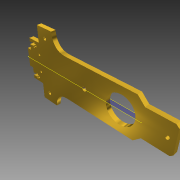
# Autodesk Inventor part: tiltColumnStepperSide02_RB01
Saved by Autodesk Inventor 2013 (Build 170138000, 138)
## iProperties
Created: 2014-06-14
Part Number: tiltColumnStepperSide02_RB01
Material: Gold
Document SubType Name: Modeling
Designer: Byron
Density: 19.3 g/cm^3
Mass: 1131.92 g
Surface Area: 227.905 cm^2
Volume: 58.6488 cm^3
Author: Byron
Autodesk Inventor part; units mm, degrees
ref_plane "YZ Plane" through (0, 0, 0) normal (1, 0, 0) x (0, 1, 0)
ref_plane "XZ Plane" through (0, 0, 0) normal (0, 1, 0) x (-1, 0, 0)
ref_plane "XY Plane" through (0, 0, 0) normal (0, 0, 1) x (1, 0, 0)
sketch "Sketch1" plane through (0, 0, 0) normal (0, 0, 1) x (1, 0, 0)
  line L0 (-21.15, 15.4985) -> (-15.4985, 21.15)
  line L1 (-15.4985, 21.15) -> (15.4985, 21.15)
  line L2 (15.4985, 21.15) -> (21.15, 15.4985)
  line L3 (21.15, 15.4985) -> (21.15, -15.4985)
  line L4 (21.15, -15.4985) -> (15.4985, -21.15)
  line L5 (15.4985, -21.15) -> (-15.4985, -21.15)
  line L6 (-15.4985, -21.15) -> (-21.15, -15.4985)
  line L7 (-21.15, -15.4985) -> (-21.15, 15.4985)
  line L8 (28.575, -18.574) -> (28.575, 18.574)
  line L9 (28.575, 18.574) -> (18.574, 28.575)
  line L10 (18.574, 28.575) -> (-18.574, 28.575)
  line L11 (-18.574, 28.575) -> (-28.575, 18.574)
  line L12 (-28.575, 18.574) -> (-28.575, -18.574)
  line L13 (-28.575, -18.574) -> (-18.574, -28.575)
  line L14 (-18.574, -28.575) -> (18.574, -28.575)
  line L15 (18.574, -28.575) -> (28.575, -18.574)
  line L16 (-18.574, -28.575) -> (-145.574, -28.575)
  line L17 (-145.574, -28.575) -> (-145.574, 28.575)
  line L18 (-145.574, 28.575) -> (-18.574, 28.575)
  line L19 (-18.574, 28.575) -> (-18.574, -28.575)
  circle A0 centre (0, 0) radius 11
  point P0 (0, 0)
  dimension "d0" = 127
  dimension "d1" = 57.15
  dimension "d2" = 57.15
  constraints: 40 end point, 2 parallel, 1 centre point, 1 horizontal, 1 perpendicular, 7 other
  measures "d0" distance of L17.end L18.end
  measures "d1" distance between parallel lines of L10 L14
  measures "d2" distance of L16.end L17.end
extrude "Extrusion1" add sketch "Sketch1" along normal blind 6.35 contours L7 L6 L19 L13 L12 L11 L0 | L0 L19 L6 L7 | L19 L10 L9 L8 L15 L14 L6 L5 L4 L3 L2 L1 L0 | L0 L1 L2 L3 L4 L5 L6 L19 | L11 L12 L13 L16 L17 L18 | A0
sketch "Sketch2" plane through (0, 0, 0) normal (0, 0, -1) x (-1, 0, 0)
  line L0 (130.4486, -16.3493) -> (130.4486, -9.9993) projected
  line L1 (126.7402, -9.9993) -> (126.7402, -16.3493) projected
  line L2 (130.4486, 9.0507) -> (130.4486, 15.4007) projected
  line L3 (126.7402, 15.4007) -> (126.7402, 9.0507) projected
  line L4 (126.7402, -12.7) -> (130.4486, -12.7) construction
  line L5 (126.7402, 12.7) -> (130.4486, 12.7) construction
  circle A0 centre (128.5944, -12.065) radius 1.8542
  circle A1 centre (128.5944, 12.065) radius 1.8542
  line L6 (-18.574, 28.575) -> (145.574, 28.575) projected
  line L7 (145.574, -28.575) -> (-18.574, -28.575) projected
  line L8 (242.583, -12.065) -> (-73.768, -12.065)
  dimension "d5" = 3.7084
  dimension "d6" = 3.7084
  dimension "d13" = 16.51
  dimension "d14" = 16.51
  dimension "d15" = 16.51
  constraints: 6 end point, 2 centre point, 1 horizontal, 2 other
  measures "d5" diameter of A0
  measures "d6" diameter of A1
  measures "d13" distance between parallel lines of L7 L8
  measures "d14" distance from line of L7 A0.centre
  measures "d15" distance from line of L6 A1.centre
extrude "Extrusion2" cut sketch "Sketch2" against normal through all
sketch "Sketch3" plane through (0, 0, 0) normal (0, 0, -1) x (-1, 0, 0)
  line L0 (145.574, 28.575) -> (145.574, -28.575) projected
  line L1 (139.224, -24.0792) -> (145.574, -24.0792) projected
  line L2 (145.574, -28.575) -> (145.574, -24.0792) projected
  line L3 (-18.574, -28.575) -> (145.574, -28.575) projected
  line L4 (-28.575, -18.574) -> (-18.574, -28.575) projected
  line L5 (-28.575, 18.574) -> (-28.575, -18.574) projected
  line L6 (-18.574, 28.575) -> (-28.575, 18.574) projected
  line L7 (145.574, 28.575) -> (-18.574, 28.575) projected
  line L8 (145.574, 24.0792) -> (145.574, 28.575) projected
  line L9 (145.574, 24.0792) -> (139.224, 24.0792) projected
  line L10 (139.224, 24.0792) -> (139.224, 26.162) projected
  line L11 (139.224, 26.162) -> (136.43, 26.162) projected
  line L12 (136.43, 26.162) -> (136.43, 24.0792) projected
  line L13 (136.43, 24.0792) -> (132.874, 24.0792) projected
  line L14 (132.874, 24.0792) -> (132.874, 20.3708) projected
  line L15 (132.874, 20.3708) -> (136.43, 20.3708) projected
  line L16 (136.43, 20.3708) -> (136.43, 18.288) projected
  line L17 (136.43, 18.288) -> (139.224, 18.288) projected
  line L18 (139.224, 18.288) -> (139.224, 20.3708) projected
  line L19 (139.224, 20.3708) -> (145.574, 20.3708) projected
  line L20 (145.574, -20.3708) -> (145.574, 20.3708) projected
  line L21 (145.574, -20.3708) -> (139.224, -20.3708) projected
  line L22 (139.224, -20.3708) -> (139.224, -18.288) projected
  line L23 (139.224, -18.288) -> (136.43, -18.288) projected
  line L24 (136.43, -18.288) -> (136.43, -20.3708) projected
  line L25 (136.43, -20.3708) -> (132.874, -20.3708) projected
  line L26 (132.874, -20.3708) -> (132.874, -24.0792) projected
  line L27 (132.874, -24.0792) -> (136.43, -24.0792) projected
  line L28 (136.43, -24.0792) -> (136.43, -26.162) projected
  line L29 (136.43, -26.162) -> (139.224, -26.162) projected
  line L30 (139.224, -26.162) -> (139.224, -24.0792) projected
  circle A0 centre (128.5944, 12.7) radius 1.8542 projected
  circle A1 centre (128.5944, -12.7) radius 1.8542 projected
  circle A2 centre (-15.5, -15.5) radius 2 projected
  circle A3 centre (15.5, -15.5) radius 2 projected
  circle A4 centre (-15.5, 15.5) radius 2 projected
  circle A5 centre (15.5, 15.5) radius 2 projected
  circle A6 centre (0, 0) radius 11 projected
extrude "Extrusion3" cut sketch "Sketch3" against normal through all contours L0 L19 L18 L17 L16 L15 L14 L13 L12 L11 L10 L9 | L0 L1 L30 L29 L28 L27 L26 L25 L24 L23 L22 L21
sketch "Sketch4" plane through (0, 0, 0) normal (0, 0, -1) x (-1, 0, 0)
  circle A0 centre (0, 0) radius 11 projected
  circle A1 centre (0, 0) radius 19.05 projected
  point P0 (0, 0)
  dimension "d24" = 38.1
  dimension "d25" = 22
  measures "d24" diameter of A1
  measures "d25" diameter of A0
extrude "Extrusion4" cut sketch "Sketch4" against normal through all contours A0 | A1
sketch "Sketch5" plane through (-145.574, -20.3708, 0) normal (-1, 0, 0) x (0, 0, 1)
  line L0 (0, 40.7416) -> (0, 0) projected
  line L1 (0, 33.0708) -> (0, 7.6708) projected
  line L2 (0, 7.6708) -> (6.35, 7.6708) projected
  line L3 (6.35, 7.6708) -> (6.35, 33.0708) projected
  line L4 (6.35, 33.0708) -> (0, 33.0708) projected
  point P0 (0, 20.3708)
extrude "Extrusion5" add sketch "Sketch5" along normal blind 6.35
sketch "Sketch6" plane through (0, 0, 6.35) normal (0, 0, 1) x (1, 0, 0)
  line L0 (-145.574, 28.575) -> (18.574, 28.575) projected
  circle A0 centre (-114.3, 38.1) radius 2.5146 projected
  circle A1 centre (-114.3, -38.1) radius 2.5146 projected
  line L1 (0, 50.8) -> (-127, 50.8) projected
  line L2 (-127, 50.8) -> (-127, -50.8) projected
  line L3 (-127, -50.8) -> (0, -50.8) projected
  line L4 (-127, 50.8) -> (-101.6, 50.8)
  line L5 (-101.6, 28.575) -> (-127, 28.575)
  line L6 (-127, 28.575) -> (-127, 50.8)
  spline S0 degree 4 poles (-101.6, 50.8) (-101.4278, 37.6809) (-93.5766, 28.9843) (-86.3032, 28.7086) (-77.2189, 28.575) knots 0 0 0 0 0 1 1 1 1 1
  line L7 (-101.6678, 55.9666) -> (-101.5322, 45.6334) construction
  arc A2 (-101.3699, 54.8975) -> (-101.2624, 46.71) centre (-71.935, 51.1893) ccw construction
  line L8 (-81.6682, 28.6405) -> (-72.7695, 28.5095) construction
  arc A3 (-80.7781, 28.6371) -> (-73.6593, 28.5323) centre (-67.6175, 681.2105) ccw construction
  line L9 (-151.924, 0) -> (28.575, 0) construction
  line L10 (0, -50.8) -> (-127, -50.8)
  line L11 (-101.6, -50.8) -> (-101.6, -28.575)
  line L12 (-127, -28.575) -> (-127, -50.8)
  spline S1 degree 4 poles (-101.6, -50.8) (-101.4278, -37.6809) (-93.5766, -28.9843) (-86.3032, -28.7086) (-77.2189, -28.575) knots 0 0 0 0 0 1 1 1 1 1
  line L13 (-101.6678, -55.9666) -> (-101.5322, -45.6334) construction
  arc A4 (-101.2624, -46.71) -> (-101.3699, -54.8975) centre (-71.935, -51.1893) ccw construction
  line L14 (-81.6682, -28.6405) -> (-72.7695, -28.5095) construction
  arc A5 (-73.6593, -28.5323) -> (-80.7781, -28.6371) centre (-67.6175, -681.2105) ccw construction
  line L15 (-77.2189, 28.575) -> (-101.6, 28.5129)
  point P0 (-91.9655, 31.5993)
  point P1 (-91.9655, -31.5993)
  constraints: 23 end point, 18 symmetric about line, 6 midpoint, 4 centre point, 4 point on circle, 3 point on line, 1 horizontal, 1 parallel, 15 other
extrude "Extrusion6" add sketch "Sketch6" against normal blind 6.35 contours L2 L1 S0 L0
ref_plane "Work Plane1" through (-145.574, 0, 0) normal (0, -1, 0) x (1, 0, 0)
mirror "Mirror1" about plane through (-145.574, 0, 0) normal (0, -1, 0) of "Extrusion6"
sketch "Sketch7" plane through (0, 0, 0) normal (0, 0, -1) x (-1, 0, 0)
  line L0 (-28.575, 18.574) -> (-18.574, 28.575)
  line L1 (-18.574, -28.575) -> (-28.575, -18.574)
  line L2 (-28.575, -18.574) -> (-28.575, 18.574)
  line L3 (-60.325, -19.2943) -> (-48.1038, -19.2943)
  line L4 (-63.5, -16.1193) -> (-60.325, -19.2943)
  line L5 (-63.5, 16.1193) -> (-63.5, -16.1193)
  line L6 (-60.325, 19.2943) -> (-63.5, 16.1193)
  line L7 (-48.1038, 19.2943) -> (-60.325, 19.2943)
  line L8 (-48.1038, 19.2943) -> (-27.8548, 19.2943)
  line L9 (-48.1038, -19.2943) -> (-27.8548, -19.2943)
  circle A0 centre (-54.61, 0) radius 2.5146
extrude "Extrusion7" add sketch "Sketch7" against normal blind 6.35
sketch "Sketch8" plane through (0, 0, 0) normal (0, 0, -1) x (-1, 0, 0)
  circle A0 centre (50.8, 0) radius 3.175 projected
extrude "Extrusion8" cut sketch "Sketch8" against normal through all
equation "\"d2\" = d1"
equation "\"d14\" = d13"
equation "\"d15\" = d14"
body "Solid1"
